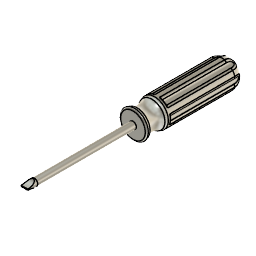
Oct24_Screwdriver (Autodesk Fusion 360 design; units mm, degrees)
part number: 2025-10-24-16-08-04-888
part number: 2025-10-24-16-08-41-428
part number: 2025-10-24-16-08-45-767
part number: 2025-10-24-16-42-45-800
Autodesk Fusion 360 part; units mm, degrees
sketch "Sketch1" plane through (0, 0, 0) normal (0, 1, 0) x (1, 0, 0) in component "Handle"
  circle A0 centre (0, 0) radius 14
  dimension "d1" = 28
  constraint coincident A0.centre origin
  measures "d1" diameter of A0
extrude "Extrude1" add sketch "Sketch1" along normal blind 100 makes body 1 in component "Handle"
sketch "Sketch2" plane through (0, 100, 0) normal (0, 1, 0) x (-1, 0, 0) in component "Handle"
  circle A0 centre (0, 0) radius 14
  circle A1 centre (-7.3986, 11.8853) radius 3
  dimension "d4" = 6
  constraint coincident A0 A1.centre
  measures "d4" diameter of A1
extrude "Extrude2" cut sketch "Sketch2" against normal blind 75 contours A0 A1 picked at (-6.8627, 11.0129) bodies 1 in component "Handle"
pattern_circular "C-Pattern1" count 6 over 360 about axis through (0, 1.75, 0) along (0, 1, 0) of "Extrude2" in component "Handle"
sketch "Sketch3" plane through (0, 0, 0) normal (1, 0, 0) x (0, 1, 0) in component "Handle"
  line L0 (0, -14) -> (100, -14)
  line L1 (100, 14) -> (0, 14)
  arc A0 (3, 14) -> (20.3205, 14) centre (11.6603, 25) ccw
  dimension "d9" = 14
  dimension "d10" = 3
  dimension "d11" = 11
  constraint coincident L1 A0.start
  constraint coincident L1 A0.end
  measures "d9" radius of A0
  measures "d10" distance of L1.end A0.start
  measures "d11" vertical distance of L1.end A0.centre
revolve "Revolve1" cut sketch "Sketch3" angle 360 about axis through (0, 1.75, 0) along (0, 1, 0) bodies 1 in component "Handle"
sketch "Sketch4" plane through (0, 0, 0) normal (0, -1, 0) x (1, 0, 0) in component "Handle"
  circle A0 centre (0, 0) radius 14
  circle A1 centre (0, 0) radius 3.5
  dimension "d13" = 7
  constraint coincident A0.centre A1.centre
  measures "d13" diameter of A1
extrude "Extrude3" cut sketch "Sketch4" against normal blind 50 contours A1 bodies 1 in component "Handle"
fillet "Fillet1" radius 5 2 edges at (-13.0526, 3, -5.0626) (-13.0526, 20.3205, 5.0626) on bodies 1 in component "Handle"
fillet "Fillet1" radius 1.5 1 edges at (-13.0526, 0, 5.0626) on bodies 1 in component "Handle"
fillet "Fillet1" radius 10 6 edges at (12.35, 100, 6.5937) (0.4647, 100, 13.9923) (-11.8853, 100, 7.3986) (-12.35, 100, -6.5937) (-0.4647, 100, -13.9923) (11.8853, 100, -7.3986) on bodies 1 in component "Handle"
fillet "Fillet2" radius 2 18 edges at (4.6965, 57.5, 13.1887) (5.706, 97.138, 9.4085) (9.7609, 57.5, 10.0362) (13.77, 57.5, 2.5271) (11.062, 97.0788, 0.178) (13.572, 57.5, -3.4351) (-9.0735, 57.5, 10.6617) (-5.2913, 97.1383, 9.6475) (-3.8111, 57.5, 13.4713) (9.0735, 57.5, -10.6617) (5.2913, 97.1383, -9.6475) (3.8111, 57.5, -13.4713) (-4.6965, 57.5, -13.1887) (-5.706, 97.138, -9.4085) (-9.7609, 57.5, -10.0362) (-13.77, 57.5, -2.5271) (-11.062, 97.0788, -0.178) (-13.572, 57.5, 3.4351) on bodies 1 in component "Handle"
fillet "Fillet2" radius 1 6 edges at (-13.9923, 25, 0.4647) (-7.3986, 25, -11.8853) (-6.5937, 25, 12.35) (7.3986, 25, 11.8853) (13.9923, 25, -0.4647) (6.5937, 25, -12.35) on bodies 1 in component "Handle"
sketch "Sketch1 (2)" plane through (0, 50, 0) normal (0, -1, 0) x (1, 0, 0) in component "Shank"
  circle A0 centre (0, 0) radius 3.5
  circle A1 centre (0, 0) radius 3.5
extrude "Extrude1'" add sketch "Sketch1 (2)" along normal blind 150 separate body makes body 2 in component "Shank"
sketch "Sketch1 (3)" plane through (0, -100, 0) normal (0, -1, 0) x (1, 0, 0) in component "Tip"
  circle A0 centre (0, 0) radius 3.5
extrude "Extrude1''" add sketch "Sketch1 (3)" along normal blind 10 separate body makes body 3 in component "Tip"
sketch "Sketch2 (2)" plane through (0, 0, 0) normal (1, 0, 0) x (0, 1, 0) in component "Tip"
  line L0 (-100, 3.5) -> (-110, 3.5)
  line L1 (-110, -3.5) -> (-100, -3.5)
  arc A0 (-110, 0.5) -> (-101, 3.5) centre (-110.3322, 16.4966) ccw
  line L2 (-110, 0.5) -> (-110, 3.5)
  point P0 (-110, 0)
  dimension "d30" = 0.5
  dimension "d31" = 9
  dimension "d32" = 16
  constraint coincident L0 A0.end
  constraint vertical L0.end A0.start
  constraint coincident L0.end L2.end
  measures "d30" distance of A0.start P0
  measures "d31" distance of L0.end A0.end
  measures "d32" radius of A0
extrude "Extrude2'" cut sketch "Sketch2 (2)" along normal through all and the other way through all bodies 3 in component "Tip"
mirror "Mirror1" about plane through (0, 0, 0) normal (0, 0, 1) of "Extrude2'" in component "Tip"
component "Handle" placed x (1, 0, 0) y (0, 1, 0) z (0, 0, 1) at (0, 0, 0)
component "Shank" placed x (1, 0, 0) y (0, 1, 0) z (0, 0, 1) at (0, 0, 0)
component "Tip" placed x (1, 0, 0) y (0, 1, 0) z (0, 0, 1) at (0, 0, 0)
